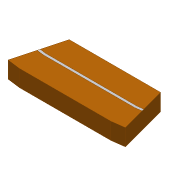
# Autodesk Inventor part: Hill 1
Saved by Autodesk Inventor 2015 SP1 (Build 190203100, 203)
## iProperties
Created: 2015-08-24
Part Number: Hill 1
Material: 一般
Document SubType Name: Modeling
Designer: nobuhiro
Density: 1 g/cm^3
Appearance: オレンジ
Author: nobuhiro
Autodesk Inventor part; units mm, degrees
ref_plane "YZ Plane" through (0, 0, 0) normal (1, 0, 0) x (0, 1, 0)
ref_plane "XZ Plane" through (0, 0, 0) normal (0, 1, 0) x (-1, 0, 0)
ref_plane "XY Plane" through (0, 0, 0) normal (0, 0, 1) x (1, 0, 0)
sketch "スケッチ1" plane through (0, 0, 0) normal (0, 0, 1) x (1, 0, 0)
  line L0 (-550, 300) -> (550, 300)
  line L1 (550, 300) -> (550, -300)
  line L2 (550, -300) -> (-550, -300)
  line L3 (-550, -300) -> (-550, 300)
  line L4 (-550, 300) -> (-705.2914, -279.5555)
  line L5 (-705.2914, -279.5555) -> (-550, -300)
  line L6 (-550, 0) -> (-627.6457, 10.2223)
  line L7 (550, 300) -> (705.2914, -279.5555)
  line L8 (705.2914, -279.5555) -> (550, -300)
  point P0 (0, 0)
  point P1 (0, 300)
  point P2 (550, 0)
  dimension "d0" = 600
  dimension "d1" = 1100
  dimension "d2" = 15
  dimension "d3" = 600
  dimension "d4" = 600
  dimension "d5" = 15
  constraints: 18 end point, 4 midpoint, 2 parallel, 1 horizontal, 1 horizontal alignment, 1 perpendicular, 1 vertical alignment
  measures "d0" distance between parallel lines of L0 L2
  measures "d1" distance of L0.start L0.end
  measures "d2" angle of L3 L4
  measures "d3" distance of L0.start L4.end
  measures "d4" distance of L0.end L7.end
  measures "d5" angle of L7 L1
extrude "押し出し1" add sketch "スケッチ1" along normal blind 200
sketch "スケッチ2" plane through (0, 0, 200) normal (0, 0, 1) x (1, 0, 0)
  line L0 (-550, 300) -> (-705.2914, -279.5555) projected
  line L1 (705.2914, -279.5555) -> (550, 300) projected
  line L2 (550, 300) -> (-550, 300) projected
  line L3 (-550, 300) -> (-550, -300)
  line L4 (550, -300) -> (550, 300)
  line L5 (-627.6457, 10.2223) -> (-550, 0)
  line L6 (550, 0) -> (-550, 0)
  line L7 (550, 0) -> (627.6457, 10.2223)
  line L8 (-631.5615, -4.3917) -> (-550.9832, -15)
  line L9 (-550.9832, -15) -> (550.9832, -15)
  line L10 (550.9832, -15) -> (631.5615, -4.3917)
  line L11 (-623.7299, 24.8362) -> (-549.0168, 15)
  line L12 (-549.0168, 15) -> (549.0168, 15)
  line L13 (549.0168, 15) -> (623.7299, 24.8362)
  line L14 (631.5615, -4.3917) -> (623.7299, 24.8362)
  line L15 (-631.5615, -4.3917) -> (-623.7299, 24.8362)
  point P0 (0, 0)
  dimension "d8" = 15
  dimension "d10" = 15
  dimension "d11" = 30
  dimension "d12" = 15
  dimension "d13" = 30
  dimension "d14" = 15
  constraints: 26 end point, 5 point on line, 4 midpoint, 2 collinear, 1 perpendicular, 1 vertical
  measures "d8" distance between parallel lines of L5 L8
  measures "d10" distance between parallel lines of L5 L11
  measures "d11" distance between parallel lines of L12 L9
  measures "d12" distance between parallel lines of L6 L9
  measures "d13" distance between parallel lines of L13 L10
  measures "d14" distance between parallel lines of L10 L7
extrude "押し出し2" add sketch "スケッチ2" along normal blind 0.1 contours L11 L3 L5 L0 | L11 L12 L13 L4 L6 L3 | L5 L3 L9 L8 L0 | L1 L7 L4 L13 | L6 L4 L9 L3 | L1 L10 L9 L4 L7
